Autodesk Inventor part; units mm, degrees
(part 2 of 4)
  line L475 (32.326357, -111.758962) -> (30.323034, -113.917658) construction
  line L476 (30.323034, -113.917658) -> (27.543531, -113.917658) construction
  line L477 (27.543531, -113.917658) -> (24.750075, -113.917658) construction
  line L478 (24.750075, -113.917658) -> (22.732455, -111.758962) construction
  line L479 (22.732455, -111.758962) -> (22.732455, -108.965506) construction
  line L480 (22.732455, -108.965506) -> (22.732455, -106.17205) construction
  line L481 (22.732455, -106.17205) -> (24.750075, -104.027478) construction
  line L482 (24.750075, -104.027478) -> (27.543531, -104.027478) construction
  spline S59 degree 3 poles (24.256221, -108.965506) (24.256221, -110.700801) (25.497833, -112.224566) (27.529406, -112.224566) (29.561151, -112.224566) (30.802591, -110.700801) (30.802591, -108.965506) (30.802591, -107.244164) (29.561151, -105.720571) (27.529406, -105.720571) (25.497833, -105.720571) (24.256221, -107.244164) (24.256221, -108.965506) knots 0 0 0 0 1 1 1 2 2 2 3 3 3 4 4 4 4
  line L483 (24.256221, -108.965506) -> (24.256221, -110.700801) construction
  line L484 (24.256221, -110.700801) -> (25.497833, -112.224566) construction
  line L485 (25.497833, -112.224566) -> (27.529406, -112.224566) construction
  line L486 (27.529406, -112.224566) -> (29.561151, -112.224566) construction
  line L487 (29.561151, -112.224566) -> (30.802591, -110.700801) construction
  line L488 (30.802591, -110.700801) -> (30.802591, -108.965506) construction
  line L489 (30.802591, -108.965506) -> (30.802591, -107.244164) construction
  line L490 (30.802591, -107.244164) -> (29.561151, -105.720571) construction
  line L491 (29.561151, -105.720571) -> (27.529406, -105.720571) construction
  line L492 (27.529406, -105.720571) -> (25.497833, -105.720571) construction
  line L493 (25.497833, -105.720571) -> (24.256221, -107.244164) construction
  line L494 (24.256221, -107.244164) -> (24.256221, -108.965506) construction
  line L495 (26.330168, -120.973731) -> (24.086722, -123.216832)
  spline S60 degree 3 poles (24.086722, -123.216832) (23.917568, -123.400456) (23.748069, -123.485205) (23.53654, -123.485205) (23.169638, -123.485205) (22.788955, -123.146553) (22.788955, -122.6949) (22.788955, -122.440997) (22.901609, -122.271843) (23.085233, -122.102344) knots 1 1 1 1 2 2 2 3 3 3 4 4 4 4
  line L496 (24.086722, -123.216832) -> (23.917568, -123.400456) construction
  line L497 (23.917568, -123.400456) -> (23.748069, -123.485205) construction
  line L498 (23.748069, -123.485205) -> (23.53654, -123.485205) construction
  line L499 (23.53654, -123.485205) -> (23.169638, -123.485205) construction
  line L500 (23.169638, -123.485205) -> (22.788955, -123.146553) construction
  line L501 (22.788955, -123.146553) -> (22.788955, -122.6949) construction
  line L502 (22.788955, -122.6949) -> (22.788955, -122.440997) construction
  line L503 (22.788955, -122.440997) -> (22.901609, -122.271843) construction
  line L504 (22.901609, -122.271843) -> (23.085233, -122.102344) construction
  line L505 (23.085233, -122.102344) -> (26.118639, -119.196062)
  line L506 (26.118639, -119.196062) -> (26.118639, -117.615968)
  line L507 (26.118639, -117.615968) -> (23.480041, -117.615968)
  spline S61 degree 3 poles (23.480041, -117.615968) (23.056983, -117.615968) (22.788955, -117.29144) (22.788955, -116.839961) (22.788955, -116.388481) (23.056983, -116.063953) (23.480041, -116.063953) knots 7 7 7 7 8 8 8 9 9 9 9
  line L508 (23.480041, -117.615968) -> (23.056983, -117.615968) construction
  line L509 (23.056983, -117.615968) -> (22.788955, -117.29144) construction
  line L510 (22.788955, -117.29144) -> (22.788955, -116.839961) construction
  line L511 (22.788955, -116.839961) -> (22.788955, -116.388481) construction
  line L512 (22.788955, -116.388481) -> (23.056983, -116.063953) construction
  line L513 (23.056983, -116.063953) -> (23.480041, -116.063953) construction
  line L514 (23.480041, -116.063953) -> (31.508147, -116.063953)
  spline S62 degree 3 poles (31.508147, -116.063953) (31.917252, -116.063953) (32.171155, -116.317856) (32.171155, -116.769336) knots 10 10 10 10 11 11 11 11
  line L515 (31.508147, -116.063953) -> (31.917252, -116.063953) construction
  line L516 (31.917252, -116.063953) -> (32.171155, -116.317856) construction
  line L517 (32.171155, -116.317856) -> (32.171155, -116.769336) construction
  line L518 (32.171155, -116.769336) -> (32.171155, -119.675619)
  spline S63 degree 3 poles (32.171155, -119.675619) (32.171155, -122.271843) (30.760389, -123.358081) (29.236623, -123.358081) (28.093713, -123.358081) (26.711196, -122.652526) (26.330168, -120.973731) knots 12 12 12 12 13 13 13 14 14 14 14
  line L519 (32.171155, -119.675619) -> (32.171155, -122.271843) construction
  line L520 (32.171155, -122.271843) -> (30.760389, -123.358081) construction
  line L521 (30.760389, -123.358081) -> (29.236623, -123.358081) construction
  line L522 (29.236623, -123.358081) -> (28.093713, -123.358081) construction
  line L523 (28.093713, -123.358081) -> (26.711196, -122.652526) construction
  line L524 (26.711196, -122.652526) -> (26.330168, -120.973731) construction
  spline S64 degree 3 poles (27.515281, -119.562964) (27.515281, -121.114635) (28.248914, -121.665161) (29.137749, -121.665161) (30.012631, -121.665161) (30.746264, -121.114635) (30.746264, -119.562964) knots 0 0 0 0 1 1 1 2 2 2 2
  line L525 (27.515281, -119.562964) -> (27.515281, -121.114635) construction
  line L526 (27.515281, -121.114635) -> (28.248914, -121.665161) construction
  line L527 (28.248914, -121.665161) -> (29.137749, -121.665161) construction
  line L528 (29.137749, -121.665161) -> (30.012631, -121.665161) construction
  line L529 (30.012631, -121.665161) -> (30.746264, -121.114635) construction
  line L530 (30.746264, -121.114635) -> (30.746264, -119.562964) construction
  line L531 (30.746264, -119.562964) -> (30.746264, -117.89795)
  spline S65 degree 3 poles (30.746264, -117.89795) (30.746264, -117.700546) (30.661515, -117.615968) (30.421736, -117.615968) knots 3 3 3 3 4 4 4 4
  line L532 (30.746264, -117.89795) -> (30.746264, -117.700546) construction
  line L533 (30.746264, -117.700546) -> (30.661515, -117.615968) construction
  line L534 (30.661515, -117.615968) -> (30.421736, -117.615968) construction
  line L535 (30.421736, -117.615968) -> (27.515281, -117.615968)
  line L536 (27.515281, -117.615968) -> (27.515281, -119.562964)
  line L537 (29.77268, -133.080485) -> (26.795773, -131.048913)
  spline S66 degree 3 poles (26.795773, -131.048913) (26.372543, -130.766759) (26.203217, -130.540761) (26.203217, -130.160078) (26.203217, -129.793175) (26.372543, -129.581646) (26.795773, -129.285368) knots 1 1 1 1 2 2 2 3 3 3 3
  line L538 (26.795773, -131.048913) -> (26.372543, -130.766759) construction
  line L539 (26.372543, -130.766759) -> (26.203217, -130.540761) construction
  line L540 (26.203217, -130.540761) -> (26.203217, -130.160078) construction
  line L541 (26.203217, -130.160078) -> (26.203217, -129.793175) construction
  line L542 (26.203217, -129.793175) -> (26.372543, -129.581646) construction
  line L543 (26.372543, -129.581646) -> (26.795773, -129.285368) construction
  line L544 (26.795773, -129.285368) -> (29.77268, -127.253451)
  line L545 (29.77268, -127.253451) -> (29.77268, -127.211421)
  line L546 (29.77268, -127.211421) -> (23.480041, -127.211421)
  spline S67 degree 3 poles (23.480041, -127.211421) (23.056983, -127.211421) (22.788955, -126.886893) (22.788955, -126.435241) (22.788955, -125.983933) (23.056983, -125.659405) (23.480041, -125.659405) knots 6 6 6 6 7 7 7 8 8 8 8
  line L547 (23.480041, -127.211421) -> (23.056983, -127.211421) construction
  line L548 (23.056983, -127.211421) -> (22.788955, -126.886893) construction
  line L549 (22.788955, -126.886893) -> (22.788955, -126.435241) construction
  line L550 (22.788955, -126.435241) -> (22.788955, -125.983933) construction
  line L551 (22.788955, -125.983933) -> (23.056983, -125.659405) construction
  line L552 (23.056983, -125.659405) -> (23.480041, -125.659405) construction
  line L553 (23.480041, -125.659405) -> (31.352945, -125.659405)
  spline S68 degree 3 poles (31.352945, -125.659405) (31.903127, -125.659405) (32.255905, -126.054213) (32.255905, -126.57649) knots 9 9 9 9 10 10 10 10
  line L554 (31.352945, -125.659405) -> (31.903127, -125.659405) construction
  line L555 (31.903127, -125.659405) -> (32.255905, -126.054213) construction
  line L556 (32.255905, -126.054213) -> (32.255905, -126.57649) construction
  line L557 (32.255905, -126.57649) -> (32.255905, -126.689144)
  spline S69 degree 3 poles (32.255905, -126.689144) (32.255905, -127.225546) (31.931377, -127.563854) (31.508147, -127.846007) knots 11 11 11 11 12 12 12 12
  line L558 (32.255905, -126.689144) -> (32.255905, -127.225546) construction
  line L559 (32.255905, -127.225546) -> (31.931377, -127.563854) construction
  line L560 (31.931377, -127.563854) -> (31.508147, -127.846007) construction
  line L561 (31.508147, -127.846007) -> (28.065635, -130.202453)
  line L562 (28.065635, -130.202453) -> (28.065635, -130.216577)
  line L563 (28.065635, -130.216577) -> (31.522272, -132.558553)
  spline S70 degree 3 poles (31.522272, -132.558553) (31.931377, -132.840707) (32.255905, -133.108735) (32.255905, -133.644792) knots 15 15 15 15 16 16 16 16
  line L564 (31.522272, -132.558553) -> (31.931377, -132.840707) construction
  line L565 (31.931377, -132.840707) -> (32.255905, -133.108735) construction
  line L566 (32.255905, -133.108735) -> (32.255905, -133.644792) construction
  line L567 (32.255905, -133.644792) -> (32.255905, -133.757791)
  spline S71 degree 3 poles (32.255905, -133.757791) (32.255905, -134.265598) (31.903127, -134.660751) (31.352945, -134.660751) knots 17 17 17 17 18 18 18 18
  line L568 (32.255905, -133.757791) -> (32.255905, -134.265598) construction
  line L569 (32.255905, -134.265598) -> (31.903127, -134.660751) construction
  line L570 (31.903127, -134.660751) -> (31.352945, -134.660751) construction
  line L571 (31.352945, -134.660751) -> (23.480041, -134.660751)
  spline S72 degree 3 poles (23.480041, -134.660751) (23.056983, -134.660751) (22.788955, -134.336223) (22.788955, -133.884571) (22.788955, -133.433263) (23.056983, -133.108735) (23.480041, -133.108735) knots 19 19 19 19 20 20 20 21 21 21 21
  line L572 (23.480041, -134.660751) -> (23.056983, -134.660751) construction
  line L573 (23.056983, -134.660751) -> (22.788955, -134.336223) construction
  line L574 (22.788955, -134.336223) -> (22.788955, -133.884571) construction
  line L575 (22.788955, -133.884571) -> (22.788955, -133.433263) construction
  line L576 (22.788955, -133.433263) -> (23.056983, -133.108735) construction
  line L577 (23.056983, -133.108735) -> (23.480041, -133.108735) construction
  line L578 (23.480041, -133.108735) -> (29.77268, -133.108735)
  line L579 (29.77268, -133.108735) -> (29.77268, -133.080485)
  spline S73 degree 3 poles (24.213846, -141.321843) (24.213846, -142.831484) (25.243757, -143.776818) (26.852273, -143.776818) knots 0 0 0 0 1 1 1 1
  line L580 (24.213846, -141.321843) -> (24.213846, -142.831484) construction
  line L581 (24.213846, -142.831484) -> (25.243757, -143.776818) construction
  line L582 (25.243757, -143.776818) -> (26.852273, -143.776818) construction
  line L583 (26.852273, -143.776818) -> (31.578599, -143.776818)
  spline S74 degree 3 poles (31.578599, -143.776818) (31.987876, -143.776818) (32.27003, -144.101001) (32.27003, -144.552653) (32.27003, -145.003961) (31.987876, -145.328489) (31.578599, -145.328489) knots 2 2 2 2 3 3 3 4 4 4 4
  line L584 (31.578599, -143.776818) -> (31.987876, -143.776818) construction
  line L585 (31.987876, -143.776818) -> (32.27003, -144.101001) construction
  line L586 (32.27003, -144.101001) -> (32.27003, -144.552653) construction
  line L587 (32.27003, -144.552653) -> (32.27003, -145.003961) construction
  line L588 (32.27003, -145.003961) -> (31.987876, -145.328489) construction
  line L589 (31.987876, -145.328489) -> (31.578599, -145.328489) construction
  line L590 (31.578599, -145.328489) -> (26.767523, -145.328489)
  spline S75 degree 3 poles (26.767523, -145.328489) (24.425375, -145.328489) (22.704205, -143.832973) (22.704205, -141.321843) (22.704205, -138.796243) (24.425375, -137.314852) (26.767523, -137.314852) knots 5 5 5 5 6 6 6 7 7 7 7
  line L591 (26.767523, -145.328489) -> (24.425375, -145.328489) construction
  line L592 (24.425375, -145.328489) -> (22.704205, -143.832973) construction
  line L593 (22.704205, -143.832973) -> (22.704205, -141.321843) construction
  line L594 (22.704205, -141.321843) -> (22.704205, -138.796243) construction
  line L595 (22.704205, -138.796243) -> (24.425375, -137.314852) construction
  line L596 (24.425375, -137.314852) -> (26.767523, -137.314852) construction
  line L597 (26.767523, -137.314852) -> (31.578599, -137.314852)
  spline S76 degree 3 poles (31.578599, -137.314852) (31.987876, -137.314852) (32.27003, -137.63938) (32.27003, -138.090688) (32.27003, -138.54234) (31.987876, -138.866868) (31.578599, -138.866868) knots 8 8 8 8 9 9 9 10 10 10 10
  line L598 (31.578599, -137.314852) -> (31.987876, -137.314852) construction
  line L599 (31.987876, -137.314852) -> (32.27003, -137.63938) construction
  line L600 (32.27003, -137.63938) -> (32.27003, -138.090688) construction
  line L601 (32.27003, -138.090688) -> (32.27003, -138.54234) construction
  line L602 (32.27003, -138.54234) -> (31.987876, -138.866868) construction
  line L603 (31.987876, -138.866868) -> (31.578599, -138.866868) construction
  line L604 (31.578599, -138.866868) -> (26.852273, -138.866868)
  spline S77 degree 3 poles (26.852273, -138.866868) (25.257882, -138.866868) (24.213846, -139.798077) (24.213846, -141.321843) knots 11 11 11 11 12 12 12 12
  line L605 (26.852273, -138.866868) -> (25.257882, -138.866868) construction
  line L606 (25.257882, -138.866868) -> (24.213846, -139.798077) construction
  line L607 (24.213846, -139.798077) -> (24.213846, -141.321843) construction
  spline S78 degree 3 poles (32.255905, -148.75877) (32.255905, -149.210422) (31.987876, -149.53495) (31.578599, -149.53495) knots 0 0 0 0 1 1 1 1
  line L608 (32.255905, -148.75877) -> (32.255905, -149.210422) construction
  line L609 (32.255905, -149.210422) -> (31.987876, -149.53495) construction
  line L610 (31.987876, -149.53495) -> (31.578599, -149.53495) construction
  line L611 (31.578599, -149.53495) -> (24.651201, -149.53495)
  spline S79 degree 3 poles (24.651201, -149.53495) (24.397125, -149.53495) (24.326501, -149.619355) (24.326501, -149.817104) knots 2 2 2 2 3 3 3 3
  line L612 (24.651201, -149.53495) -> (24.397125, -149.53495) construction
  line L613 (24.397125, -149.53495) -> (24.326501, -149.619355) construction
  line L614 (24.326501, -149.619355) -> (24.326501, -149.817104) construction
  line L615 (24.326501, -149.817104) -> (24.326501, -153.936749)
  spline S80 degree 3 poles (24.326501, -153.936749) (24.326501, -154.402181) (24.058472, -154.684335) (23.607165, -154.684335) (23.155513, -154.684335) (22.887484, -154.402181) (22.887484, -153.936749) knots 4 4 4 4 5 5 5 6 6 6 6
  line L616 (24.326501, -153.936749) -> (24.326501, -154.402181) construction
  line L617 (24.326501, -154.402181) -> (24.058472, -154.684335) construction
  line L618 (24.058472, -154.684335) -> (23.607165, -154.684335) construction
  line L619 (23.607165, -154.684335) -> (23.155513, -154.684335) construction
  line L620 (23.155513, -154.684335) -> (22.887484, -154.402181) construction
  line L621 (22.887484, -154.402181) -> (22.887484, -153.936749) construction
  line L622 (22.887484, -153.936749) -> (22.887484, -148.744645)
  spline S81 degree 3 poles (22.887484, -148.744645) (22.887484, -148.279213) (23.141388, -147.982935) (23.607165, -147.982935) knots 7 7 7 7 8 8 8 8
  line L623 (22.887484, -148.744645) -> (22.887484, -148.279213) construction
  line L624 (22.887484, -148.279213) -> (23.141388, -147.982935) construction
  line L625 (23.141388, -147.982935) -> (23.607165, -147.982935) construction
  line L626 (23.607165, -147.982935) -> (31.578599, -147.982935)
  spline S82 degree 3 poles (31.578599, -147.982935) (31.987876, -147.982935) (32.255905, -148.307463) (32.255905, -148.75877) knots 9 9 9 9 10 10 10 10
  line L627 (31.578599, -147.982935) -> (31.987876, -147.982935) construction
  line L628 (31.987876, -147.982935) -> (32.255905, -148.307463) construction
  line L629 (32.255905, -148.307463) -> (32.255905, -148.75877) construction
  line L630 (25.15918, -157.831774) -> (23.367386, -157.098313)
  spline S83 degree 3 poles (23.367386, -157.098313) (22.986359, -156.942939) (22.788955, -156.703161) (22.788955, -156.336258) (22.788955, -155.88495) (23.085233, -155.574547) (23.494166, -155.546298) knots 1 1 1 1 2 2 2 3 3 3 3
  line L631 (23.367386, -157.098313) -> (22.986359, -156.942939) construction
  line L632 (22.986359, -156.942939) -> (22.788955, -156.703161) construction
  line L633 (22.788955, -156.703161) -> (22.788955, -156.336258) construction
  line L634 (22.788955, -156.336258) -> (22.788955, -155.88495) construction
  line L635 (22.788955, -155.88495) -> (23.085233, -155.574547) construction
  line L636 (23.085233, -155.574547) -> (23.494166, -155.546298) construction
  spline S84 degree 3 poles (23.494166, -155.546298) (23.677789, -155.532173) (23.846944, -155.588672) (24.044348, -155.673422) knots 3 3 3 3 4 4 4 4
  line L637 (23.494166, -155.546298) -> (23.677789, -155.532173) construction
  line L638 (23.677789, -155.532173) -> (23.846944, -155.588672) construction
  line L639 (23.846944, -155.588672) -> (24.044348, -155.673422) construction
  line L640 (24.044348, -155.673422) -> (31.169494, -158.636204)
  spline S85 degree 3 poles (31.169494, -158.636204) (31.959627, -158.946607) (32.255905, -159.369664) (32.255905, -160.004596) knots 5 5 5 5 6 6 6 6
  line L641 (31.169494, -158.636204) -> (31.959627, -158.946607) construction
  line L642 (31.959627, -158.946607) -> (32.255905, -159.369664) construction
  line L643 (32.255905, -159.369664) -> (32.255905, -160.004596) construction
  line L644 (32.255905, -160.004596) -> (32.255905, -160.10347)
  spline S86 degree 3 poles (32.255905, -160.10347) (32.255905, -160.752526) (31.959627, -161.161459) (31.169494, -161.485987) knots 7 7 7 7 8 8 8 8
  line L645 (32.255905, -160.10347) -> (32.255905, -160.752526) construction
  line L646 (32.255905, -160.752526) -> (31.959627, -161.161459) construction
  line L647 (31.959627, -161.161459) -> (31.169494, -161.485987) construction
  line L648 (31.169494, -161.485987) -> (23.988192, -164.448769)
  spline S87 degree 3 poles (23.988192, -164.448769) (23.804569, -164.519393) (23.64954, -164.561768) (23.53654, -164.561768) (23.099358, -164.561768) (22.788955, -164.20899) (22.788955, -163.743558) (22.788955, -163.404905) (23.000484, -163.122752) (23.381511, -162.967378) knots 9 9 9 9 10 10 10 11 11 11 12 12 12 12
  line L649 (23.988192, -164.448769) -> (23.804569, -164.519393) construction
  line L650 (23.804569, -164.519393) -> (23.64954, -164.561768) construction
  line L651 (23.64954, -164.561768) -> (23.53654, -164.561768) construction
  line L652 (23.53654, -164.561768) -> (23.099358, -164.561768) construction
  line L653 (23.099358, -164.561768) -> (22.788955, -164.20899) construction
  line L654 (22.788955, -164.20899) -> (22.788955, -163.743558) construction
  line L655 (22.788955, -163.743558) -> (22.788955, -163.404905) construction
  line L656 (22.788955, -163.404905) -> (23.000484, -163.122752) construction
  line L657 (23.000484, -163.122752) -> (23.381511, -162.967378) construction
  line L658 (23.381511, -162.967378) -> (25.15918, -162.248042)
  line L659 (25.15918, -162.248042) -> (25.15918, -157.831774)
  line L660 (26.570119, -161.69786) -> (30.703889, -160.07522)
  line L661 (30.703889, -160.07522) -> (30.703889, -160.032845)
  line L662 (30.703889, -160.032845) -> (26.570119, -158.368175)
  line L663 (26.570119, -158.368175) -> (26.570119, -161.69786)
  spline S88 degree 3 poles (31.451647, -164.295117) (31.903127, -164.295117) (32.171155, -164.591396) (32.171155, -165.057173) knots 0 0 0 0 1 1 1 1
  line L664 (31.451647, -164.295117) -> (31.903127, -164.295117) construction
  line L665 (31.903127, -164.295117) -> (32.171155, -164.591396) construction
  line L666 (32.171155, -164.591396) -> (32.171155, -165.057173) construction
  line L667 (32.171155, -165.057173) -> (32.171155, -172.266724)
  spline S89 degree 3 poles (32.171155, -172.266724) (32.171155, -172.732156) (31.903127, -173.01431) (31.451647, -173.01431) (31.014292, -173.01431) (30.746264, -172.732156) (30.746264, -172.266724) knots 2 2 2 2 3 3 3 4 4 4 4
  line L668 (32.171155, -172.266724) -> (32.171155, -172.732156) construction
  line L669 (32.171155, -172.732156) -> (31.903127, -173.01431) construction
  line L670 (31.903127, -173.01431) -> (31.451647, -173.01431) construction
  line L671 (31.451647, -173.01431) -> (31.014292, -173.01431) construction
  line L672 (31.014292, -173.01431) -> (30.746264, -172.732156) construction
  line L673 (30.746264, -172.732156) -> (30.746264, -172.266724) construction
  line L674 (30.746264, -172.266724) -> (30.746264, -169.444846)
  line L675 (30.746264, -169.444846) -> (23.480041, -169.444846)
  spline S90 degree 3 poles (23.480041, -169.444846) (23.071108, -169.444846) (22.788955, -169.120318) (22.788955, -168.669011) (22.788955, -168.217359) (23.071108, -167.892831) (23.480041, -167.892831) knots 6 6 6 6 7 7 7 8 8 8 8
  line L676 (23.480041, -169.444846) -> (23.071108, -169.444846) construction
  line L677 (23.071108, -169.444846) -> (22.788955, -169.120318) construction
  line L678 (22.788955, -169.120318) -> (22.788955, -168.669011) construction
  line L679 (22.788955, -168.669011) -> (22.788955, -168.217359) construction
  line L680 (22.788955, -168.217359) -> (23.071108, -167.892831) construction
  line L681 (23.071108, -167.892831) -> (23.480041, -167.892831) construction
  line L682 (23.480041, -167.892831) -> (30.746264, -167.892831)
  line L683 (30.746264, -167.892831) -> (30.746264, -165.043048)
  spline S91 degree 3 poles (30.746264, -165.043048) (30.746264, -164.591396) (31.014292, -164.295117) (31.451647, -164.295117) knots 10 10 10 10 11 11 11 11
  line L684 (30.746264, -165.043048) -> (30.746264, -164.591396) construction
  line L685 (30.746264, -164.591396) -> (31.014292, -164.295117) construction
  line L686 (31.014292, -164.295117) -> (31.451647, -164.295117) construction
  spline S92 degree 3 poles (32.27003, -175.372133) (32.27003, -175.823441) (31.987876, -176.147969) (31.578599, -176.147969) knots 0 0 0 0 1 1 1 1
  line L687 (32.27003, -175.372133) -> (32.27003, -175.823441) construction
  line L688 (32.27003, -175.823441) -> (31.987876, -176.147969) construction
  line L689 (31.987876, -176.147969) -> (31.578599, -176.147969) construction
  line L690 (31.578599, -176.147969) -> (23.480041, -176.147969)
  spline S93 degree 3 poles (23.480041, -176.147969) (23.071108, -176.147969) (22.788955, -175.823441) (22.788955, -175.372133) (22.788955, -174.920481) (23.071108, -174.595953) (23.480041, -174.595953) knots 2 2 2 2 3 3 3 4 4 4 4
  line L691 (23.480041, -176.147969) -> (23.071108, -176.147969) construction
  line L692 (23.071108, -176.147969) -> (22.788955, -175.823441) construction
  line L693 (22.788955, -175.823441) -> (22.788955, -175.372133) construction
  line L694 (22.788955, -175.372133) -> (22.788955, -174.920481) construction
  line L695 (22.788955, -174.920481) -> (23.071108, -174.595953) construction
  line L696 (23.071108, -174.595953) -> (23.480041, -174.595953) construction
  line L697 (23.480041, -174.595953) -> (31.578599, -174.595953)
  spline S94 degree 3 poles (31.578599, -174.595953) (31.987876, -174.595953) (32.27003, -174.920481) (32.27003, -175.372133) knots 5 5 5 5 6 6 6 6
  line L698 (31.578599, -174.595953) -> (31.987876, -174.595953) construction
  line L699 (31.987876, -174.595953) -> (32.27003, -174.920481) construction
  line L700 (32.27003, -174.920481) -> (32.27003, -175.372133) construction
  spline S95 degree 3 poles (27.543531, -178.279105) (30.323034, -178.279105) (32.326357, -180.423677) (32.326357, -183.217304) (32.326357, -186.010932) (30.323034, -188.169629) (27.543531, -188.169629) (24.750075, -188.169629) (22.732455, -186.010932) (22.732455, -183.217304) (22.732455, -180.423677) (24.750075, -178.279105) (27.543531, -178.279105) knots 0 0 0 0 1 1 1 2 2 2 3 3 3 4 4 4 4
  line L701 (27.543531, -178.279105) -> (30.323034, -178.279105) construction
  line L702 (30.323034, -178.279105) -> (32.326357, -180.423677) construction
  line L703 (32.326357, -180.423677) -> (32.326357, -183.217304) construction
  line L704 (32.326357, -183.217304) -> (32.326357, -186.010932) construction
  line L705 (32.326357, -186.010932) -> (30.323034, -188.169629) construction
  line L706 (30.323034, -188.169629) -> (27.543531, -188.169629) construction
  line L707 (27.543531, -188.169629) -> (24.750075, -188.169629) construction
  line L708 (24.750075, -188.169629) -> (22.732455, -186.010932) construction
  line L709 (22.732455, -186.010932) -> (22.732455, -183.217304) construction
  line L710 (22.732455, -183.217304) -> (22.732455, -180.423677) construction
  line L711 (22.732455, -180.423677) -> (24.750075, -178.279105) construction
  line L712 (24.750075, -178.279105) -> (27.543531, -178.279105) construction
  spline S96 degree 3 poles (24.256221, -183.217304) (24.256221, -184.952599) (25.497833, -186.476365) (27.529406, -186.476365) (29.561151, -186.476365) (30.802591, -184.952599) (30.802591, -183.217304) (30.802591, -181.496135) (29.561151, -179.972369) (27.529406, -179.972369) (25.497833, -179.972369) (24.256221, -181.496135) (24.256221, -183.217304) knots 0 0 0 0 1 1 1 2 2 2 3 3 3 4 4 4 4
  line L713 (24.256221, -183.217304) -> (24.256221, -184.952599) construction
  line L714 (24.256221, -184.952599) -> (25.497833, -186.476365) construction
  line L715 (25.497833, -186.476365) -> (27.529406, -186.476365) construction
  line L716 (27.529406, -186.476365) -> (29.561151, -186.476365) construction
  line L717 (29.561151, -186.476365) -> (30.802591, -184.952599) construction
  line L718 (30.802591, -184.952599) -> (30.802591, -183.217304) construction
  line L719 (30.802591, -183.217304) -> (30.802591, -181.496135) construction
  line L720 (30.802591, -181.496135) -> (29.561151, -179.972369) construction
  line L721 (29.561151, -179.972369) -> (27.529406, -179.972369) construction
  line L722 (27.529406, -179.972369) -> (25.497833, -179.972369) construction
  line L723 (25.497833, -179.972369) -> (24.256221, -181.496135) construction
  line L724 (24.256221, -181.496135) -> (24.256221, -183.217304) construction
  line L725 (22.788955, -197.567505) -> (22.788955, -197.51135)
  spline S97 degree 3 poles (22.788955, -197.51135) (22.788955, -197.031448) (23.000484, -196.721045) (23.494166, -196.368267) knots 1 1 1 1 2 2 2 2
  line L726 (22.788955, -197.51135) -> (22.788955, -197.031448) construction
  line L727 (22.788955, -197.031448) -> (23.000484, -196.721045) construction
  line L728 (23.000484, -196.721045) -> (23.494166, -196.368267) construction
  line L729 (23.494166, -196.368267) -> (29.80093, -191.867595)
  line L730 (29.80093, -191.867595) -> (23.480041, -191.867595)
  spline S98 degree 3 poles (23.480041, -191.867595) (23.071108, -191.867595) (22.788955, -191.543067) (22.788955, -191.091759) (22.788955, -190.640107) (23.071108, -190.315579) (23.480041, -190.315579) knots 4 4 4 4 5 5 5 6 6 6 6
  line L731 (23.480041, -191.867595) -> (23.071108, -191.867595) construction
  line L732 (23.071108, -191.867595) -> (22.788955, -191.543067) construction
  line L733 (22.788955, -191.543067) -> (22.788955, -191.091759) construction
  line L734 (22.788955, -191.091759) -> (22.788955, -190.640107) construction
  line L735 (22.788955, -190.640107) -> (23.071108, -190.315579) construction
  line L736 (23.071108, -190.315579) -> (23.480041, -190.315579) construction
  line L737 (23.480041, -190.315579) -> (31.324696, -190.315579)
  spline S99 degree 3 poles (31.324696, -190.315579) (31.889002, -190.315579) (32.255905, -190.696607) (32.255905, -191.176509) knots 7 7 7 7 8 8 8 8
  line L738 (31.324696, -190.315579) -> (31.889002, -190.315579) construction
  line L739 (31.889002, -190.315579) -> (32.255905, -190.696607) construction
  line L740 (32.255905, -190.696607) -> (32.255905, -191.176509) construction
  line L741 (32.255905, -191.176509) -> (32.255905, -191.260913)
  spline S100 degree 3 poles (32.255905, -191.260913) (32.255905, -191.740815) (32.086578, -191.994719) (31.479897, -192.446026) knots 9 9 9 9 10 10 10 10
  line L742 (32.255905, -191.260913) -> (32.255905, -191.740815) construction
  line L743 (32.255905, -191.740815) -> (32.086578, -191.994719) construction
  line L744 (32.086578, -191.994719) -> (31.479897, -192.446026) construction
  line L745 (31.479897, -192.446026) -> (25.356757, -196.946699)
  line L746 (25.356757, -196.946699) -> (31.578599, -196.946699)
  spline S101 degree 3 poles (31.578599, -196.946699) (31.987876, -196.946699) (32.27003, -197.271227) (32.27003, -197.722879) (32.27003, -198.174187) (31.987876, -198.498714) (31.578599, -198.498714) knots 12 12 12 12 13 13 13 14 14 14 14
  line L747 (31.578599, -196.946699) -> (31.987876, -196.946699) construction
  line L748 (31.987876, -196.946699) -> (32.27003, -197.271227) construction
  line L749 (32.27003, -197.271227) -> (32.27003, -197.722879) construction
  line L750 (32.27003, -197.722879) -> (32.27003, -198.174187) construction
  line L751 (32.27003, -198.174187) -> (31.987876, -198.498714) construction
  line L752 (31.987876, -198.498714) -> (31.578599, -198.498714) construction
  line L753 (31.578599, -198.498714) -> (23.62129, -198.498714)
  spline S102 degree 3 poles (23.62129, -198.498714) (23.127263, -198.498714) (22.788955, -198.061532) (22.788955, -197.567505) knots 15 15 15 15 16 16 16 16
  line L754 (23.62129, -198.498714) -> (23.127263, -198.498714) construction
  line L755 (23.127263, -198.498714) -> (22.788955, -198.061532) construction
  line L756 (22.788955, -198.061532) -> (22.788955, -197.567505) construction
  spline S103 degree 3 poles (15.322399, -97.296279) (15.322399, -97.747758) (15.054371, -98.072286) (14.645093, -98.072286) knots 0 0 0 0 1 1 1 1
  line L757 (15.322399, -97.296279) -> (15.322399, -97.747758) construction
  line L758 (15.322399, -97.747758) -> (15.054371, -98.072286) construction
  line L759 (15.054371, -98.072286) -> (14.645093, -98.072286) construction
  line L760 (14.645093, -98.072286) -> (7.717695, -98.072286)
  spline S104 degree 3 poles (7.717695, -98.072286) (7.463792, -98.072286) (7.393167, -98.156863) (7.393167, -98.35444) knots 2 2 2 2 3 3 3 3
  line L761 (7.717695, -98.072286) -> (7.463792, -98.072286) construction
  line L762 (7.463792, -98.072286) -> (7.393167, -98.156863) construction
  line L763 (7.393167, -98.156863) -> (7.393167, -98.35444) construction
  line L764 (7.393167, -98.35444) -> (7.393167, -102.474085)
  spline S105 degree 3 poles (7.393167, -102.474085) (7.393167, -102.939689) (7.125139, -103.221843) (6.673832, -103.221843) (6.22218, -103.221843) (5.954151, -102.939689) (5.954151, -102.474085) knots 4 4 4 4 5 5 5 6 6 6 6
  line L765 (7.393167, -102.474085) -> (7.393167, -102.939689) construction
  line L766 (7.393167, -102.939689) -> (7.125139, -103.221843) construction
  line L767 (7.125139, -103.221843) -> (6.673832, -103.221843) construction
  line L768 (6.673832, -103.221843) -> (6.22218, -103.221843) construction
  line L769 (6.22218, -103.221843) -> (5.954151, -102.939689) construction
  line L770 (5.954151, -102.939689) -> (5.954151, -102.474085) construction
  line L771 (5.954151, -102.474085) -> (5.954151, -97.282154)
  spline S106 degree 3 poles (5.954151, -97.282154) (5.954151, -96.816549) (6.208055, -96.520271) (6.673832, -96.520271) knots 7 7 7 7 8 8 8 8
  line L772 (5.954151, -97.282154) -> (5.954151, -96.816549) construction
  line L773 (5.954151, -96.816549) -> (6.208055, -96.520271) construction
  line L774 (6.208055, -96.520271) -> (6.673832, -96.520271) construction
  line L775 (6.673832, -96.520271) -> (14.645093, -96.520271)
  spline S107 degree 3 poles (14.645093, -96.520271) (15.054371, -96.520271) (15.322399, -96.844799) (15.322399, -97.296279) knots 9 9 9 9 10 10 10 10
  line L776 (14.645093, -96.520271) -> (15.054371, -96.520271) construction
  line L777 (15.054371, -96.520271) -> (15.322399, -96.844799) construction
  line L778 (15.322399, -96.844799) -> (15.322399, -97.296279) construction
  line L779 (8.225847, -106.369282) -> (6.434053, -105.635649)
  spline S108 degree 3 poles (6.434053, -105.635649) (6.053025, -105.480447) (5.855277, -105.240669) (5.855277, -104.873766) (5.855277, -104.422286) (6.1519, -104.111883) (6.560832, -104.083633) knots 1 1 1 1 2 2 2 3 3 3 3
  line L780 (6.434053, -105.635649) -> (6.053025, -105.480447) construction
  line L781 (6.053025, -105.480447) -> (5.855277, -105.240669) construction
  line L782 (5.855277, -105.240669) -> (5.855277, -104.873766) construction
  line L783 (5.855277, -104.873766) -> (5.855277, -104.422286) construction
  line L784 (5.855277, -104.422286) -> (6.1519, -104.111883) construction
  line L785 (6.1519, -104.111883) -> (6.560832, -104.083633) construction
  spline S109 degree 3 poles (6.560832, -104.083633) (6.744456, -104.069681) (6.91361, -104.126008) (7.111014, -104.210757) knots 3 3 3 3 4 4 4 4
  line L786 (6.560832, -104.083633) -> (6.744456, -104.069681) construction
  line L787 (6.744456, -104.069681) -> (6.91361, -104.126008) construction
  line L788 (6.91361, -104.126008) -> (7.111014, -104.210757) construction
  line L789 (7.111014, -104.210757) -> (14.236161, -107.17354)
  spline S110 degree 3 poles (14.236161, -107.17354) (15.026121, -107.483943) (15.322399, -107.907173) (15.322399, -108.542104) knots 5 5 5 5 6 6 6 6
  line L790 (14.236161, -107.17354) -> (15.026121, -107.483943) construction
  line L791 (15.026121, -107.483943) -> (15.322399, -107.907173) construction
  line L792 (15.322399, -107.907173) -> (15.322399, -108.542104) construction
  line L793 (15.322399, -108.542104) -> (15.322399, -108.640806)
  spline S111 degree 3 poles (15.322399, -108.640806) (15.322399, -109.289862) (15.026121, -109.698967) (14.236161, -110.023495) knots 7 7 7 7 8 8 8 8
  line L794 (15.322399, -108.640806) -> (15.322399, -109.289862) construction
  line L795 (15.322399, -109.289862) -> (15.026121, -109.698967) construction
  line L796 (15.026121, -109.698967) -> (14.236161, -110.023495) construction
  line L797 (14.236161, -110.023495) -> (7.054859, -112.986277)
  spline S112 degree 3 poles (7.054859, -112.986277) (6.871236, -113.056901) (6.716206, -113.099276) (6.603207, -113.099276) (6.166024, -113.099276) (5.855277, -112.746498) (5.855277, -112.280894) (5.855277, -111.942241) (6.06715, -111.660087) (6.448178, -111.504886) knots 9 9 9 9 10 10 10 11 11 11 12 12 12 12
  line L798 (7.054859, -112.986277) -> (6.871236, -113.056901) construction
  line L799 (6.871236, -113.056901) -> (6.716206, -113.099276) construction
  line L800 (6.716206, -113.099276) -> (6.603207, -113.099276) construction
  line L801 (6.603207, -113.099276) -> (6.166024, -113.099276) construction
  line L802 (6.166024, -113.099276) -> (5.855277, -112.746498) construction
  line L803 (5.855277, -112.746498) -> (5.855277, -112.280894) construction
  line L804 (5.855277, -112.280894) -> (5.855277, -111.942241) construction
  line L805 (5.855277, -111.942241) -> (6.06715, -111.660087) construction
  line L806 (6.06715, -111.660087) -> (6.448178, -111.504886) construction
  line L807 (6.448178, -111.504886) -> (8.225847, -110.785378)
  line L808 (8.225847, -110.785378) -> (8.225847, -106.369282)
  line L809 (9.636614, -110.235196) -> (13.770384, -108.612556)
  line L810 (13.770384, -108.612556) -> (13.770384, -108.570354)
  line L811 (13.770384, -108.570354) -> (9.636614, -106.905511)
  line L812 (9.636614, -106.905511) -> (9.636614, -110.235196)
  line L813 (6.631457, -114.991322) -> (14.574814, -114.991322)
  spline S113 degree 3 poles (14.574814, -114.991322) (14.983746, -114.991322) (15.23765, -115.245226) (15.23765, -115.696706) knots 1 1 1 1 2 2 2 2
  line L814 (14.574814, -114.991322) -> (14.983746, -114.991322) construction
  line L815 (14.983746, -114.991322) -> (15.23765, -115.245226) construction
  line L816 (15.23765, -115.245226) -> (15.23765, -115.696706) construction
  line L817 (15.23765, -115.696706) -> (15.23765, -118.70169)
  spline S114 degree 3 poles (15.23765, -118.70169) (15.23765, -120.959261) (14.123162, -122.102) (12.599396, -122.102) (11.668186, -122.102) (10.864101, -121.509443) (10.553698, -120.747733) knots 3 3 3 3 4 4 4 5 5 5 5
  line L818 (15.23765, -118.70169) -> (15.23765, -120.959261) construction
  line L819 (15.23765, -120.959261) -> (14.123162, -122.102) construction
  line L820 (14.123162, -122.102) -> (12.599396, -122.102) construction
  line L821 (12.599396, -122.102) -> (11.668186, -122.102) construction
  line L822 (11.668186, -122.102) -> (10.864101, -121.509443) construction
  line L823 (10.864101, -121.509443) -> (10.553698, -120.747733) construction
  spline S115 degree 3 poles (10.553698, -120.747733) (10.215045, -121.819846) (9.35446, -122.355903) (8.493876, -122.355903) (7.040734, -122.355903) (5.954151, -121.19904) (5.954151, -119.068593) knots 5 5 5 5 6 6 6 7 7 7 7
  line L824 (10.553698, -120.747733) -> (10.215045, -121.819846) construction
  line L825 (10.215045, -121.819846) -> (9.35446, -122.355903) construction
  line L826 (9.35446, -122.355903) -> (8.493876, -122.355903) construction
  line L827 (8.493876, -122.355903) -> (7.040734, -122.355903) construction
  line L828 (7.040734, -122.355903) -> (5.954151, -121.19904) construction
  line L829 (5.954151, -121.19904) -> (5.954151, -119.068593) construction
  line L830 (5.954151, -119.068593) -> (5.954151, -115.696706)
  spline S116 degree 3 poles (5.954151, -115.696706) (5.954151, -115.245226) (6.208055, -114.991322) (6.631457, -114.991322) knots 8 8 8 8 9 9 9 9
  line L831 (5.954151, -115.696706) -> (5.954151, -115.245226) construction
  line L832 (5.954151, -115.245226) -> (6.208055, -114.991322) construction
  line L833 (6.208055, -114.991322) -> (6.631457, -114.991322) construction
  spline S117 degree 3 poles (11.089755, -118.800565) (11.089755, -119.830648) (11.541407, -120.493484) (12.430242, -120.493484) (13.319076, -120.493484) (13.812758, -119.816523) (13.812758, -118.589036) knots 0 0 0 0 1 1 1 2 2 2 2
  line L834 (11.089755, -118.800565) -> (11.089755, -119.830648) construction
  line L835 (11.089755, -119.830648) -> (11.541407, -120.493484) construction
  line L836 (11.541407, -120.493484) -> (12.430242, -120.493484) construction
  line L837 (12.430242, -120.493484) -> (13.319076, -120.493484) construction
  line L838 (13.319076, -120.493484) -> (13.812758, -119.816523) construction
  line L839 (13.812758, -119.816523) -> (13.812758, -118.589036) construction
  line L840 (13.812758, -118.589036) -> (13.812758, -116.825491)
  spline S118 degree 3 poles (13.812758, -116.825491) (13.812758, -116.627915) (13.728009, -116.543338) (13.48823, -116.543338) knots 3 3 3 3 4 4 4 4
  line L841 (13.812758, -116.825491) -> (13.812758, -116.627915) construction
  line L842 (13.812758, -116.627915) -> (13.728009, -116.543338) construction
  line L843 (13.728009, -116.543338) -> (13.48823, -116.543338) construction
  line L844 (13.48823, -116.543338) -> (11.089755, -116.543338)
  line L845 (11.089755, -116.543338) -> (11.089755, -118.800565)
  line L846 (7.393167, -116.825491) -> (7.393167, -118.927689)
  spline S119 degree 3 poles (7.393167, -118.927689) (7.393167, -120.183081) (7.830695, -120.733608) (8.648905, -120.733608) (9.312086, -120.733608) (9.834018, -120.211331) (9.834018, -119.181592) knots 1 1 1 1 2 2 2 3 3 3 3
  line L847 (7.393167, -118.927689) -> (7.393167, -120.183081) construction
  line L848 (7.393167, -120.183081) -> (7.830695, -120.733608) construction
  line L849 (7.830695, -120.733608) -> (8.648905, -120.733608) construction
  line L850 (8.648905, -120.733608) -> (9.312086, -120.733608) construction
  line L851 (9.312086, -120.733608) -> (9.834018, -120.211331) construction
  line L852 (9.834018, -120.211331) -> (9.834018, -119.181592) construction
  line L853 (9.834018, -119.181592) -> (9.834018, -116.543338)
  line L854 (9.834018, -116.543338) -> (7.717695, -116.543338)
  spline S120 degree 3 poles (7.717695, -116.543338) (7.463792, -116.543338) (7.393167, -116.627915) (7.393167, -116.825491) knots 5 5 5 5 6 6 6 6
  line L855 (7.717695, -116.543338) -> (7.463792, -116.543338) construction
  line L856 (7.463792, -116.543338) -> (7.393167, -116.627915) construction
  line L857 (7.393167, -116.627915) -> (7.393167, -116.825491) construction
  spline S121 degree 3 poles (10.610198, -123.853142) (13.389701, -123.853142) (15.393024, -125.997714) (15.393024, -128.790997) (15.393024, -131.584625) (13.389701, -133.743322) (10.610198, -133.743322) (7.81657, -133.743322) (5.799122, -131.584625) (5.799122, -128.790997) (5.799122, -125.997714) (7.81657, -123.853142) (10.610198, -123.853142) knots 0 0 0 0 1 1 1 2 2 2 3 3 3 4 4 4 4
  line L858 (10.610198, -123.853142) -> (13.389701, -123.853142) construction
  line L859 (13.389701, -123.853142) -> (15.393024, -125.997714) construction
  line L860 (15.393024, -125.997714) -> (15.393024, -128.790997) construction
  line L861 (15.393024, -128.790997) -> (15.393024, -131.584625) construction
  line L862 (15.393024, -131.584625) -> (13.389701, -133.743322) construction
  line L863 (13.389701, -133.743322) -> (10.610198, -133.743322) construction
  line L864 (10.610198, -133.743322) -> (7.81657, -133.743322) construction
  line L865 (7.81657, -133.743322) -> (5.799122, -131.584625) construction
  line L866 (5.799122, -131.584625) -> (5.799122, -128.790997) construction
  line L867 (5.799122, -128.790997) -> (5.799122, -125.997714) construction
  line L868 (5.799122, -125.997714) -> (7.81657, -123.853142) construction
  line L869 (7.81657, -123.853142) -> (10.610198, -123.853142) construction
  spline S122 degree 3 poles (7.322888, -128.790997) (7.322888, -130.526636) (8.5645, -132.050057) (10.596073, -132.050057) (12.627646, -132.050057) (13.869258, -130.526636) (13.869258, -128.790997) (13.869258, -127.069827) (12.627646, -125.546062) (10.596073, -125.546062) (8.5645, -125.546062) (7.322888, -127.069827) (7.322888, -128.790997) knots 0 0 0 0 1 1 1 2 2 2 3 3 3 4 4 4 4
  line L870 (7.322888, -128.790997) -> (7.322888, -130.526636) construction
  line L871 (7.322888, -130.526636) -> (8.5645, -132.050057) construction
  line L872 (8.5645, -132.050057) -> (10.596073, -132.050057) construction
  line L873 (10.596073, -132.050057) -> (12.627646, -132.050057) construction
  line L874 (12.627646, -132.050057) -> (13.869258, -130.526636) construction
  line L875 (13.869258, -130.526636) -> (13.869258, -128.790997) construction
  line L876 (13.869258, -128.790997) -> (13.869258, -127.069827) construction
  line L877 (13.869258, -127.069827) -> (12.627646, -125.546062) construction
  line L878 (12.627646, -125.546062) -> (10.596073, -125.546062) construction
  line L879 (10.596073, -125.546062) -> (8.5645, -125.546062) construction
  line L880 (8.5645, -125.546062) -> (7.322888, -127.069827) construction
  line L881 (7.322888, -127.069827) -> (7.322888, -128.790997) construction
  line L882 (9.396835, -140.799222) -> (7.153389, -143.042668)
  spline S123 degree 3 poles (7.153389, -143.042668) (6.984235, -143.225947) (6.814736, -143.310696) (6.603207, -143.310696) (6.236304, -143.310696) (5.855277, -142.972044) (5.855277, -142.520736) (5.855277, -142.266832) (5.968276, -142.097334) (6.1519, -141.92818) knots 1 1 1 1 2 2 2 3 3 3 4 4 4 4
  line L883 (7.153389, -143.042668) -> (6.984235, -143.225947) construction
  line L884 (6.984235, -143.225947) -> (6.814736, -143.310696) construction
  line L885 (6.814736, -143.310696) -> (6.603207, -143.310696) construction
  line L886 (6.603207, -143.310696) -> (6.236304, -143.310696) construction
  line L887 (6.236304, -143.310696) -> (5.855277, -142.972044) construction
  line L888 (5.855277, -142.972044) -> (5.855277, -142.520736) construction
  line L889 (5.855277, -142.520736) -> (5.855277, -142.266832) construction
  line L890 (5.855277, -142.266832) -> (5.968276, -142.097334) construction
  line L891 (5.968276, -142.097334) -> (6.1519, -141.92818) construction
  line L892 (6.1519, -141.92818) -> (9.185306, -139.021553)
  line L893 (9.185306, -139.021553) -> (9.185306, -137.441632)
  line L894 (9.185306, -137.441632) -> (6.546708, -137.441632)
  spline S124 degree 3 poles (6.546708, -137.441632) (6.12365, -137.441632) (5.855277, -137.117104) (5.855277, -136.665452) (5.855277, -136.214144) (6.12365, -135.889616) (6.546708, -135.889616) knots 7 7 7 7 8 8 8 9 9 9 9
  line L895 (6.546708, -137.441632) -> (6.12365, -137.441632) construction
  line L896 (6.12365, -137.441632) -> (5.855277, -137.117104) construction
  line L897 (5.855277, -137.117104) -> (5.855277, -136.665452) construction
  line L898 (5.855277, -136.665452) -> (5.855277, -136.214144) construction
  line L899 (5.855277, -136.214144) -> (6.12365, -135.889616) construction
  line L900 (6.12365, -135.889616) -> (6.546708, -135.889616) construction
  line L901 (6.546708, -135.889616) -> (14.574814, -135.889616)
  spline S125 degree 3 poles (14.574814, -135.889616) (14.983746, -135.889616) (15.23765, -136.14352) (15.23765, -136.594827) knots 10 10 10 10 11 11 11 11
  line L902 (14.574814, -135.889616) -> (14.983746, -135.889616) construction
  line L903 (14.983746, -135.889616) -> (15.23765, -136.14352) construction
  line L904 (15.23765, -136.14352) -> (15.23765, -136.594827) construction
  line L905 (15.23765, -136.594827) -> (15.23765, -139.501454)
  spline S126 degree 3 poles (15.23765, -139.501454) (15.23765, -142.097334) (13.826883, -143.183572) (12.303118, -143.183572) (11.160379, -143.183572) (9.777863, -142.478361) (9.396835, -140.799222) knots 12 12 12 12 13 13 13 14 14 14 14
  line L906 (15.23765, -139.501454) -> (15.23765, -142.097334) construction
  line L907 (15.23765, -142.097334) -> (13.826883, -143.183572) construction
  line L908 (13.826883, -143.183572) -> (12.303118, -143.183572) construction
  line L909 (12.303118, -143.183572) -> (11.160379, -143.183572) construction
  line L910 (11.160379, -143.183572) -> (9.777863, -142.478361) construction
  line L911 (9.777863, -142.478361) -> (9.396835, -140.799222) construction
  spline S127 degree 3 poles (10.581948, -139.388455) (10.581948, -140.940471) (11.315409, -141.490652) (12.204243, -141.490652) (13.079298, -141.490652) (13.812758, -140.940471) (13.812758, -139.388455) knots 0 0 0 0 1 1 1 2 2 2 2
  line L912 (10.581948, -139.388455) -> (10.581948, -140.940471) construction
  line L913 (10.581948, -140.940471) -> (11.315409, -141.490652) construction
  line L914 (11.315409, -141.490652) -> (12.204243, -141.490652) construction
  line L915 (12.204243, -141.490652) -> (13.079298, -141.490652) construction
  line L916 (13.079298, -141.490652) -> (13.812758, -140.940471) construction
  line L917 (13.812758, -140.940471) -> (13.812758, -139.388455) construction
  line L918 (13.812758, -139.388455) -> (13.812758, -137.723785)
  spline S128 degree 3 poles (13.812758, -137.723785) (13.812758, -137.526037) (13.728009, -137.441632) (13.48823, -137.441632) knots 3 3 3 3 4 4 4 4
  line L919 (13.812758, -137.723785) -> (13.812758, -137.526037) construction
  line L920 (13.812758, -137.526037) -> (13.728009, -137.441632) construction
  line L921 (13.728009, -137.441632) -> (13.48823, -137.441632) construction
  line L922 (13.48823, -137.441632) -> (10.581948, -137.441632)
  line L923 (10.581948, -137.441632) -> (10.581948, -139.388455)
  line L924 (8.225847, -146.938037) -> (6.434053, -146.204577)
  spline S129 degree 3 poles (6.434053, -146.204577) (6.053025, -146.049203) (5.855277, -145.809424) (5.855277, -145.442521) (5.855277, -144.991214) (6.1519, -144.680811) (6.560832, -144.652561) knots 1 1 1 1 2 2 2 3 3 3 3
  line L925 (6.434053, -146.204577) -> (6.053025, -146.049203) construction
  line L926 (6.053025, -146.049203) -> (5.855277, -145.809424) construction
  line L927 (5.855277, -145.809424) -> (5.855277, -145.442521) construction
  line L928 (5.855277, -145.442521) -> (5.855277, -144.991214) construction
  line L929 (5.855277, -144.991214) -> (6.1519, -144.680811) construction
  line L930 (6.1519, -144.680811) -> (6.560832, -144.652561) construction
  spline S130 degree 3 poles (6.560832, -144.652561) (6.744456, -144.638436) (6.91361, -144.694936) (7.111014, -144.779685) knots 3 3 3 3 4 4 4 4
  line L931 (6.560832, -144.652561) -> (6.744456, -144.638436) construction
  line L932 (6.744456, -144.638436) -> (6.91361, -144.694936) construction
  line L933 (6.91361, -144.694936) -> (7.111014, -144.779685) construction
  line L934 (7.111014, -144.779685) -> (14.236161, -147.742467)
  spline S131 degree 3 poles (14.236161, -147.742467) (15.026121, -148.05287) (15.322399, -148.475928) (15.322399, -149.110859) knots 5 5 5 5 6 6 6 6
  line L935 (14.236161, -147.742467) -> (15.026121, -148.05287) construction
  line L936 (15.026121, -148.05287) -> (15.322399, -148.475928) construction
  line L937 (15.322399, -148.475928) -> (15.322399, -149.110859) construction
  line L938 (15.322399, -149.110859) -> (15.322399, -149.209733)
  spline S132 degree 3 poles (15.322399, -149.209733) (15.322399, -149.858789) (15.026121, -150.267722) (14.236161, -150.59225) knots 7 7 7 7 8 8 8 8
  line L939 (15.322399, -149.209733) -> (15.322399, -149.858789) construction
  line L940 (15.322399, -149.858789) -> (15.026121, -150.267722) construction
  line L941 (15.026121, -150.267722) -> (14.236161, -150.59225) construction